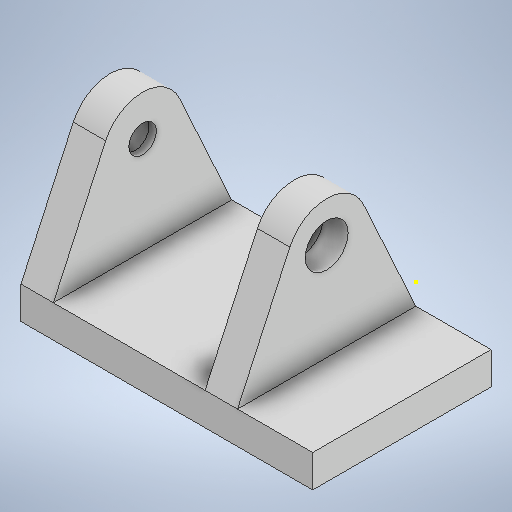
# Autodesk Inventor part: podstawa
Saved by Autodesk Inventor 2025.2 (Build 292293000, 293)
## iProperties
Created: 2025-05-19
Part Number: podstawa
Material: Ogólny
Document SubType Name: Modeling
Designer: marci
Density: 1 g/cm^3
Appearance: Domyślna
Author: marci
Autodesk Inventor part; units mm, degrees
ref_plane "YZ Plane" through (0, 0, 0) normal (1, 0, 0) x (0, 1, 0)
ref_plane "XZ Plane" through (0, 0, 0) normal (0, 1, 0) x (-1, 0, 0)
ref_plane "XY Plane" through (0, 0, 0) normal (0, 0, 1) x (1, 0, 0)
sketch "Szkic1" plane through (0, 0, 0) normal (0, 0, 1) x (1, 0, 0)
  line L0 (-172.0995, -130.735) -> (1627.9005, -130.735)
  line L1 (1627.9005, -130.735) -> (1627.9005, -330.735)
  line L2 (1627.9005, -330.735) -> (-172.0995, -330.735)
  line L3 (-172.0995, -330.735) -> (-172.0995, -130.735)
  dimension "d6" = 1800
  dimension "d7" = 200
  constraints: 8 end point, 2 parallel, 1 horizontal, 1 perpendicular
  measures "d6" distance of L1.end L2.end
  measures "d7" distance of L0.end L1.end
extrude "Wyciągnięcie proste1" add sketch "Szkic1" along normal blind 1100
sketch "Szkic2" plane through (-172.0995, -130.735, 0) normal (0, 1, 0) x (1, 0, 0)
  point P0 (172.0995, 0)
sketch "Szkic3" plane through (-172.0995, -130.735, 0) normal (0, 1, 0) x (1, 0, 0)
  line L0 (0, 0) -> (1800, 0) projected
  line L1 (0, -1100) -> (1800, -1100) projected
  line L2 (0, 0) -> (200, 0)
  line L3 (200, 0) -> (200, -1100)
  line L4 (200, -1100) -> (0, -1100)
  line L5 (0, -1100) -> (0, 0)
  line L6 (1800, 0) -> (1700, 0)
  line L7 (1700, -1100) -> (1800, -1100)
  line L8 (1336, 0) -> (1136, 0)
  line L9 (1136, 0) -> (1136, -1100)
  line L10 (1136, -1100) -> (1336, -1100)
  line L11 (1336, -1100) -> (1336, 0)
  line L12 (100, 0) -> (100, -1100)
  line L13 (1236, 0) -> (1236, -1100) construction
  point P0 (172.0995, 0)
  dimension "d10" = 200
  dimension "d15" = 200
  dimension "d21" = 936
  constraints: 24 end point, 5 parallel, 4 midpoint, 4 point on line, 3 horizontal, 2 perpendicular
  measures "d10" distance of L3.end L4.end
  measures "d15" distance of L10.end L9.end
  measures "d21" distance between parallel lines of L9 L3
extrude "Wyciągnięcie proste2" add sketch "Szkic3" along normal blind 1200 contours L0 L12 L1 L5 | L0 L3 L1 L12 | L0 L11 L1 L9
sketch "Szkic6" plane through (27.9005, -130.735, 1100) normal (1, 0, 0) x (0, 0, -1)
  line L0 (0, 1200) -> (1100, 1200) projected
  line L1 (550, 1200) -> (550, 0)
  line L2 (1100, 0) -> (0, 0) projected
  line L3 (0, 0) -> (0, 1200) projected
  line L4 (0, 600) -> (1100, 600)
  line L5 (1100, 0) -> (1100, 1200) projected
  circle A0 centre (550, 600) radius 85
  point P0 (1100, 130.735)
  dimension "d23" = 170
  constraints: 5 midpoint, 4 end point, 1 centre point
  measures "d23" diameter of A0
extrude "Wyciągnięcie proste4" cut sketch "Szkic6" along normal blind 982 and the other way blind 46 contours A0 L4 L1 | L1 L4 A0 | L4 L1 A0 | L4 A0 L1
sketch "Szkic7" plane through (1163.9005, -130.735, 1100) normal (1, 0, 0) x (0, 0, -1)
  point P0 (1100, 130.735)
sketch "Szkic8" plane through (1163.9005, -130.735, 1100) normal (1, 0, 0) x (0, 0, -1)
  circle A0 centre (550, 600) radius 85 projected
  circle A1 centre (550, 600) radius 132
  point P0 (1100, 130.735)
  dimension "d28" = 264
  constraints: 1 centre point, 1 coincident
  measures "d28" diameter of A1
extrude "Wyciągnięcie proste5" cut sketch "Szkic8" against normal up to surface (154 mm away) contours A0 | A1
sketch "Szkic9" plane through (-172.0995, -330.735, 0) normal (-1, 0, 0) x (0, 0, 1)
  circle A0 centre (550, 800) radius 85 projected
  circle A1 centre (550, 800) radius 132
  point P0 (0, 330.735)
  constraints: 1 centre point, 1 coincident
extrude "Wyciągnięcie proste6" cut sketch "Szkic9" against normal up to surface (154 mm away) contours A0 | A1
sketch "Szkic10" plane through (1163.9005, -130.735, 1100) normal (1, 0, 0) x (0, 0, -1)
  line L0 (1100, 1200) -> (0, 1200) projected
  line L1 (1100, 0) -> (0, 0) projected
  line L2 (0, -200) -> (0, 1200) projected
  circle A0 centre (550, 600) radius 250
  line L3 (0, 0) -> (322.7328, 704.1616)
  line L4 (1100, 0) -> (777.2672, 704.1616)
  line L5 (0, 0) -> (0, 1200)
  line L6 (0, 1200) -> (1100, 1200)
  line L7 (1100, -200) -> (1100, 1200) projected
  line L8 (1100, 1200) -> (1100, 0)
  point P0 (1100, 130.735)
  dimension "d33" = 500
  constraints: 10 end point, 3 collinear, 2 point on circle, 2 tangent, 1 centre point
  measures "d33" diameter of A0
extrude "Wyciągnięcie proste7" cut sketch "Szkic10" against normal through all contours L7 L4 A0 L3 L2 L0
